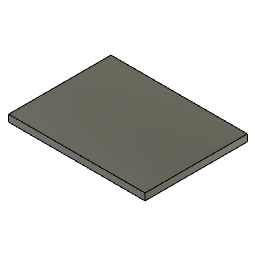
seed_container (Autodesk Fusion 360 archive; units mm, degrees)
design "plate"
Autodesk Fusion 360 part; units mm, degrees
sketch "Sketch1" plane through (0, 0, 0) normal (0, 0, 1) x (1, 0, 0)
  line L0 (0, 40) -> (40, 40)
  line L1 (40, 40) -> (40, 10)
  line L2 (40, 10) -> (0, 10)
  line L3 (0, 10) -> (0, 40)
  line L4 (42.1812, 7.8188) -> (-2.1812, 7.8188)
  line L5 (-2.1812, 7.8188) -> (-2.1812, 42.1812)
  line L6 (-2.1812, 42.1812) -> (42.1812, 42.1812)
  line L7 (42.1812, 42.1812) -> (42.1812, 7.8188)
  dimension "d1" = -2.1812
  constraint horizontal L0
  constraint vertical L1
  constraint horizontal L2
  constraint vertical L3
extrude "Extrude1" add sketch "Sketch1" along normal blind 2 contours L0 L1 L2 L3

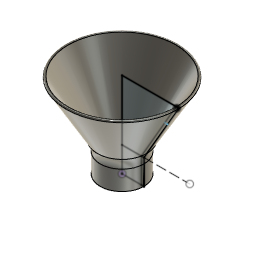
design "Salt and Pepper Grinders Funnel v2"
Autodesk Fusion 360 part; units mm, degrees
sketch "Sketch2" plane through (0, 0, 0) normal (0, 1, 0) x (1, 0, 0)
  line L0 (0, 0) -> (10.5, 0)
  line L1 (10.5, 0) -> (10.5, -12)
  line L2 (10.5, -12) -> (0, -12)
  line L3 (0, -12) -> (0, 0)
  line L4 (10.5, -12) -> (27.2, -40.9252)
  line L5 (27.2, -40.9252) -> (0, -40.9252)
  line L6 (0, -40.9252) -> (0, -12)
  line L7 (10.5, 0) -> (9.3, 0)
  line L8 (9.3, 0) -> (9.3, -12)
  line L9 (9.3, -12) -> (10.5, -12)
  line L10 (10.5, -12) -> (10.5, 0)
  line L11 (26, -40.9252) -> (9.3, -12)
  line L12 (10.5, -12) -> (32.5161, -12) construction
  line L13 (20.5641, -31.5101) -> (21.7641, -31.5101)
  circle A0 centre (26.3, -40.4056) radius 0.5196
  dimension "d2" = 10.5
  dimension "d3" = 12
  dimension "d4" = 27.2
  dimension "d21" = 1.2
  dimension "d22" = 60
  dimension "d23" = 1.2
  constraint horizontal L0
  constraint vertical L1
  constraint horizontal L2
  constraint vertical L3
  constraint coincident L0.start L3.end
  constraint perpendicular L1 L5
  constraint perpendicular L2 L6
  constraint horizontal L7
  constraint vertical L8
  constraint horizontal L9
  constraint vertical L10
  constraint coincident L2 L8.end
  constraint coincident L5 L11.start
  constraint parallel L4 L11
  constraint perpendicular L10 L12
  constraint coincident L11 L13.start
  constraint coincident L4 L13.end
  constraint horizontal L13
  constraint coincident L8.end L9.start
  constraint tangent L5 A0
  constraint tangent L4 A0
  constraint tangent L11 A0
  measures "d2" distance of L0.start L0.end
  measures "d3" distance of L0.end L1.end
  measures "d4" distance of L4.end L5.end
  measures "d21" distance of L1 L8
  measures "d22" angle of L4 L12
  measures "d23" distance of L13.start L13.end
revolve "Revolve4" add sketch "Sketch2" angle 360 about axis through (0, 0, 12) along (0, 0, -1) contours L0 L1 L2 L7 L8 L9 L10 | L2 L4 L9 L11 L13 | L4 L11 L13 A0 | A0
fillet "Fillet4" radius 10 2 edges at (-9.7894, -3.797, 12) (-8.6706, -3.363, 12)
equation "d2 = bottomOuterDiameter / 2"
equation "d3 = bottomDepth"
equation "d4 = topOuterDiameter / 2"
equation "d21 = thickness"
equation "d22 = angle"
equation "d23 = thickness"
equation "bottomOuterDiameter = 21 mm"
equation "topOuterDiameter = 54.4 mm"
equation "thickness = 1.2 mm"
equation "angle = 60 deg"
equation "bottomDepth = 12 mm"
